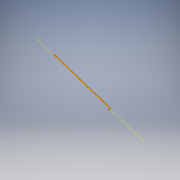
# Autodesk Inventor part: FOVStick
Saved by Autodesk Inventor 2018.2 (Build 222227000, 227)
## iProperties
Created: 2018-04-13
Part Number: FOVStick
Material: Generisch
Document SubType Name: Modeling
Designer: Nick Koch
Density: 1 g/cm^3
Appearance: Orange
Mass: 0.012 g
Surface Area: 0.32 cm^2
Volume: 0.012 cm^3
Author: Nick Koch
Autodesk Inventor part; units mm, degrees
ref_plane "YZ Plane" through (0, 0, 0) normal (1, 0, 0) x (0, 1, 0)
sketch "Skizze1" plane through (0, 0, 0) normal (0, 0, 1) x (1, 0, 0)
  line L0 (0, 0) -> (2, 0)
  line L1 (2, 0) -> (2, 2)
  line L2 (2, 2) -> (0, 2)
  line L3 (0, 2) -> (0, 0)
  dimension "d0" = 2
  dimension "d1" = 2
  constraints: 8 end point, 2 parallel, 1 horizontal, 1 perpendicular
  measures "d0" distance of L2.end L1.end
  measures "d1" distance of L1.end L0.end
extrude "Extrusion1" add sketch "Skizze1" along normal blind 3
sketch "Skizze2" plane through (0, 0, 3) normal (0, 0, 1) x (1, 0, 0)
  point P0 (0, 0)
ref_plane "Arbeitsebene1" through (0, 0, 3) normal (-0.7071068, 0.7071068, 0) x (0.7071068, 0.7071068, 0)
sketch "Skizze3" plane through (0, 0, 3) normal (-0.7071068, 0.7071068, 0) x (0.7071068, 0.7071068, 0)
  line L0 (0, 0) -> (1.4142, 0) projected
  line L1 (0, 0) -> (-112.5245, -131.9823)
  line L2 (0, 0) -> (173.439, 0) construction
  line L3 (2.8284, 3) -> (2.8284, 0) projected
  line L4 (2.8284, 0) -> (-109.6961, -131.9823)
  line L5 (2.8284, 0) -> (176.2674, 0) construction
  line L6 (-109.6961, -131.9823) -> (-112.5245, -131.9823)
  line L7 (1.4142, 0) -> (2.8284, 0) projected
  line L8 (2.8284, 0) -> (0, 0)
  point P0 (0, 3)
  dimension "d4" = 173.439
  dimension "d5" = 130.45
  dimension "d6" = 173.439
  dimension "d7" = 130.45
  constraints: 12 end point, 3 horizontal, 2 equal length
  measures "d4" distance of L0.start L1.end
  measures "d5" angle of L1 L2
  measures "d6" distance of L3.end L4.end
  measures "d7" angle of L4 L5
ref_plane "Arbeitsebene2" through (0, 0, 3) normal (0, 0.8564105, 0.5162955) x (-0.4587597, -0.4587597, 0.7609724)
sketch "Skizze4" plane through (0, 0, 3) normal (0, 0.8564105, 0.5162955) x (-0.4587597, -0.4587597, 0.7609724)
  line L0 (0, 0) -> (-0.9175, 1.7771) projected
  line L1 (0, 0) -> (-0.9175, 1.7771)
  line L2 (-0.9175, 1.7771) -> (172.5215, 1.7771)
  line L3 (172.5215, 1.7771) -> (173.439, 0)
  line L4 (173.439, 0) -> (0, 0)
  point P0 (-2.2829, -1.1787)
  dimension "d9" = 173.439
  constraints: 8 end point, 1 collinear, 1 horizontal
  measures "d9" distance of L0.end L2.end
extrude "Extrusion2" add sketch "Skizze4" along normal blind 2
sketch "Skizze5" plane through (-77.5668, -79.5668, 134.9823) normal (0.8885604, -0.2368556, 0.3928866) x (0.4587597, 0.4587597, -0.7609724)
  line L0 (172.5215, 0) -> (-0.9175, 0) projected
  line L1 (0.0005, 0) -> (1.3553, 2)
  line L2 (0, 2) -> (173.439, 2) projected
  line L3 (1.3553, 2) -> (0, 2)
  line L4 (0, 0) -> (0, 2) projected
  line L5 (0, 2) -> (0, 0)
  point P0 (174.8044, -1.5489)
  constraints: 6 end point, 2 collinear, 2 point on line
sketch "Skizze6" plane through (0, 0, 3) normal (0, -0.8564105, -0.5162955) x (0.8885604, -0.2368556, 0.3928866)
  line L0 (0, 0) -> (0, 173.439) projected
  line L1 (1.7771, 172.5215) -> (0, 173.439)
  point P0 (-1.1787, -2.2829)
  constraints: 2 end point
sketch "Skizze7" plane through (0, 1.7128, 4.0326) normal (0, 0.8564105, 0.5162955) x (0.8885604, -0.2368556, 0.3928866)
  line L0 (0, 0) -> (0, -173.439) projected
  line L1 (0, -172.1027) -> (1.781, -171.1647)
  point P0 (-1.1787, 2.2829)
  constraints: 2 end point, 1 point on line
sketch "Skizze8" plane through (0, 0, 3) normal (-0.8885604, 0.2368556, -0.3928866) x (-0.4587597, -0.4587597, 0.7609724)
  line L0 (0, 2) -> (173.439, 2) projected
  line L1 (0, 0) -> (173.439, 0) projected
  line L2 (172.1026, 2) -> (173.439, 0)
  point P0 (-2.2829, -1.5489)
  constraints: 2 end point, 1 point on line
chamfer "Fase1" distance 1.1929 distance2 2 1 edges at (-78.5668, -77.854, 136.0149) measured on face at (-25.1889, -24.8095, 48.0267)
ref_plane "Arbeitsebene3" through (2, 0, 3) normal (-1, 0, 0) x (0, 0.8564105, 0.5162955)
sketch "Skizze12" plane through (2, 0, 3) normal (-1, 0, 0) x (0, 0.8564105, 0.5162955)
  line L0 (0, 0) -> (1.7128, 1.0326) projected
  line L1 (0, 0) -> (2, 0)
  line L2 (-1.5489, 2.5692) -> (0, 0) projected
  line L3 (0, 0) -> (1.7128, 1.0326)
  line L4 (2, 0) -> (1.7128, 1.0326)
  constraints: 6 end point, 1 horizontal
extrude "Extrusion6" add sketch "Skizze12" along normal blind 2
sketch "Skizze13" plane through (0, 0, 0) normal (0, 0, -1) x (-1, 0, 0)
  line L0 (0, 2) -> (0, 0) projected
  line L1 (-2, 0) -> (-2, 2) projected
  line L2 (0, 0) -> (-2, 0)
  line L3 (-2, 0) -> (-2, 2)
  line L4 (-2, 2) -> (0, 2)
  line L5 (0, 2) -> (0, 0)
  constraints: 8 end point, 2 parallel, 1 horizontal, 1 perpendicular
extrude "Extrusion7" add sketch "Skizze13" along normal blind 2
